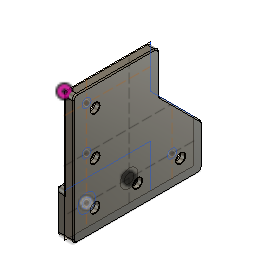
foot (Autodesk Fusion 360 design; units mm, degrees)
Autodesk Fusion 360 part; units mm, degrees
sketch "Sketch1" plane through (0, 0, 0) normal (1, 0, 0) x (0, 0, -1)
  line L0 (0, 0) -> (0, -60)
  line L1 (0, -60) -> (60, -60)
  line L2 (60, -60) -> (60, -40)
  line L3 (40, 0) -> (0, 0)
  line L4 (40, -40) -> (40, -60)
  line L5 (40, -40) -> (0, -40)
  line L6 (60, -40) -> (40, -20)
  line L7 (40, -20) -> (40, 0)
  line L8 (60, -50) -> (0, -50) construction
  line L9 (10.2088, 0) -> (10.2088, -60) construction
  line L10 (0, -9.7462) -> (40, -10) construction
  line L11 (0, -30) -> (50, -30) construction
  line L12 (49.9986, -60) -> (50, -30) construction
  line L13 (30, -60) -> (30, 0) construction
  circle A0 centre (10.2088, -9.811) radius 2.1
  circle A1 centre (10.2088, -30) radius 2.1
  circle A2 centre (10.2088, -50) radius 2.1
  circle A3 centre (30, -50) radius 2.1
  circle A4 centre (49.9991, -50) radius 2.1
  circle A5 centre (30, -50) radius 4.1
  circle A6 centre (10.2088, -50) radius 4.1
  dimension "d1" = 60
  dimension "d2" = 60
  dimension "d3" = 20
  dimension "d4" = 20
  dimension "d15" = 4.2
  dimension "d16" = 4.2
  dimension "d17" = 4.2
  dimension "d18" = 4.2
  dimension "d19" = 4.2
  dimension "d20" = 8.2
  dimension "d21" = 8.2
  constraint coincident L0.start L3.end
  constraint vertical L0
  constraint perpendicular L0 L1
  constraint perpendicular L1 L2
  constraint perpendicular L0 L3
  constraint coincident L1 L4.end
  constraint perpendicular L1 L4
  constraint coincident L0 L5.end
  constraint perpendicular L0 L5
  constraint perpendicular L3 L7
  constraint midpoint L2 L8.start
  constraint coincident L0 L8.end
  constraint perpendicular L0 L8
  constraint coincident L3 L9.start
  constraint coincident L1 L9.end
  constraint perpendicular L1 L9
  constraint coincident L0 L10.start
  constraint midpoint L7 L10.end
  constraint midpoint L0 L11.start
  constraint midpoint L6 L11.end
  constraint perpendicular L0 L11
  constraint coincident L1 L12.start
  constraint midpoint L1 L13.start
  constraint coincident L3 L13.end
  constraint perpendicular L3 L13
  constraint coincident L10 A0.centre
  constraint coincident L9 A0.centre
  constraint midpoint L9 A1.centre
  constraint coincident L8 A2.centre
  constraint coincident L9 A2.centre
  constraint midpoint L8 A3.centre
  constraint coincident L8 A4.centre
  constraint coincident L12 A4.centre
  constraint concentric A3 A5
  constraint concentric A2 A6
  measures "d1" distance of L0.start L0.end
  measures "d2" distance of L0.end L1.end
  measures "d3" distance of L1.end L2.end
  measures "d4" distance of L2.end L4.start
  measures "d15" diameter of A0
  measures "d16" diameter of A1
  measures "d17" diameter of A2
  measures "d18" diameter of A3
  measures "d19" diameter of A4
  measures "d20" diameter of A5
  measures "d21" diameter of A6
extrude "Extrude1" add sketch "Sketch1" along normal blind 4 contours L0 L1 L2 L3 L4 L5 L6 L7 | L0 L1 L4 L5 | A5 | A6
extrude "Extrude2" add sketch "Sketch1" against normal blind 5 contours L0 L1 L4 L5
chamfer "Chamfer1" distance 2 angle 45 5 edges at (0, -9.0516, -8.2509) (0, -29.2406, -8.2509) (0, -49.2406, -8.2509) (0, -49.2406, -28.0421) (0, -49.2406, -48.0412)
fillet "Fillet1" radius 2 9 edges at (2, -60, -60) (-0.5, -60, 0) (2, -40, -60) (2, -20, -40) (2, 0, -40) (2, 0, 0) (-2.5, -40, -40) (-2.5, -60, -40) (-2.5, -40, 0)
chamfer "Chamfer2" distance 0.5 angle 45 25 edges at (-5, -51.4826, -26.1775) (-5, -51.4826, -6.3862) (0, -60, -48) (0, -59.4142, -59.4142) (0, -49.4142, -60) (0, -40.0631, -59.8478) (0, -30, -50) (0, -19.9369, -40.1522) (0, -10.5858, -40) (0, -0.5858, -39.4142) (0, 0, -20) (0, -0.5858, -0.5858) (0, -22, 0) (4, -59.4142, -59.4142) (4, -49.4142, -60) (4, -40.0631, -59.8478) (4, -30, -50) (4, -19.9369, -40.1522) (4, -10.5858, -40) (4, -0.5858, -39.4142) (4, 0, -20) (4, -0.5858, -0.5858) (4, -30, 0) (4, -59.4142, -0.5858) (4, -60, -30)
chamfer "Chamfer3" distance 0.2 angle 45 5 edges at (4, -9.0516, -8.2509) (4, -29.2406, -8.2509) (4, -49.2406, -8.2509) (4, -49.2406, -28.0421) (4, -49.2406, -48.0412)
chamfer "Chamfer4" distance 2 angle 45 8 edges at (-5, -59.4142, -0.5858) (-5, -50, 0) (-5, -40.5858, -0.5858) (-5, -40, -20) (-5, -40.5858, -39.4142) (-5, -50, -40) (-5, -59.4142, -39.4142) (-5, -60, -20)
